Autodesk Inventor part; units mm, degrees
(part 2 of 2)
  spline S148 degree 2 poles (56.4799, 7.905) (55.3529, 7.905) (54.1022, 9.21) (54.1022, 10.347) knots 0 0 0 1 2 2 2
  spline S149 degree 2 poles (54.1022, 10.347) (54.1022, 11.4938) (55.3529, 12.7939) (56.4799, 12.7939) knots 0 0 0 1 2 2 2
  spline S150 degree 2 poles (56.4799, 12.7939) (57.607, 12.7939) (58.8527, 11.4889) (58.8527, 10.347) knots 0 0 0 1 2 2 2
  spline S151 degree 2 poles (57.3845, 10.3371) (57.3845, 10.7474) (57.2511, 11.2961) (57.1324, 11.4592) knots 0 0 0 1 2 2 2
  spline S152 degree 2 poles (57.1324, 11.4592) (57.0039, 11.6322) (56.6826, 11.7657) (56.4799, 11.7657) knots 0 0 0 1 2 2 2
  spline S153 degree 2 poles (56.4799, 11.7657) (56.2822, 11.7657) (55.9708, 11.6471) (55.8422, 11.479) knots 0 0 0 1 2 2 2
  spline S154 degree 2 poles (55.8422, 11.479) (55.7187, 11.3208) (55.5704, 10.7622) (55.5704, 10.3371) knots 0 0 0 1 2 2 2
  spline S155 degree 2 poles (55.5704, 10.3371) (55.5704, 9.9169) (55.7088, 9.3979) (55.8225, 9.2397) knots 0 0 0 1 2 2 2
  spline S156 degree 2 poles (55.8225, 9.2397) (55.9362, 9.0815) (56.2822, 8.9332) (56.4898, 8.9332) knots 0 0 0 1 2 2 2
  spline S157 degree 2 poles (56.4898, 8.9332) (56.6628, 8.9332) (57.0187, 9.0815) (57.1275, 9.2298) knots 0 0 0 1 2 2 2
  spline S158 degree 2 poles (57.1275, 9.2298) (57.2511, 9.4028) (57.3845, 9.9021) (57.3845, 10.3371) knots 0 0 0 1 2 2 2
  line L157 (63.9195, 8.0483) -> (62.4761, 8.0483)
  line L158 (62.4761, 8.0483) -> (62.4761, 10.3272)
  spline S159 degree 2 poles (62.4761, 10.3272) (62.4761, 10.609) (62.4316, 11.1626) (62.3723, 11.2911) knots 0 0 0 1 2 2 2
  spline S160 degree 2 poles (62.3723, 11.2911) (62.2982, 11.4493) (62.0213, 11.5828) (61.7841, 11.5828) knots 0 0 0 1 2 2 2
  spline S161 degree 2 poles (61.7841, 11.5828) (61.611, 11.5828) (61.2502, 11.4493) (61.0475, 11.306) knots 0 0 0 1 2 2 2
  line L159 (61.0475, 11.306) -> (61.0475, 8.0483)
  line L160 (61.0475, 8.0483) -> (59.614, 8.0483)
  line L161 (59.614, 8.0483) -> (59.614, 12.6505)
  line L162 (59.614, 12.6505) -> (61.0475, 12.6505)
  line L163 (61.0475, 12.6505) -> (61.0475, 12.1414)
  spline S162 degree 2 poles (61.0475, 12.1414) (61.3985, 12.438) (62.0658, 12.7741) (62.4712, 12.7741) knots 0 0 0 1 2 2 2
  spline S163 degree 2 poles (62.4712, 12.7741) (63.1731, 12.7741) (63.9195, 11.8843) (63.9195, 11.044) knots 0 0 0 1 2 2 2
  line L164 (63.9195, 11.044) -> (63.9195, 8.0483)
  spline S164 degree 2 poles (67.3403, 7.9248) (66.0353, 7.9248) (64.6462, 9.1705) (64.6462, 10.3223) knots 0 0 0 1 2 2 2
  spline S165 degree 2 poles (64.6462, 10.3223) (64.6462, 11.4493) (65.9413, 12.7939) (67.108, 12.7939) knots 0 0 0 1 2 2 2
  spline S166 degree 2 poles (67.108, 12.7939) (68.1609, 12.7939) (69.2286, 11.652) (69.2286, 10.5941) knots 0 0 0 1 2 2 2
  line L165 (69.2286, 10.5941) -> (69.2286, 10.0751)
  line L166 (69.2286, 10.0751) -> (66.0798, 10.0751)
  spline S167 degree 2 poles (66.0798, 10.0751) (66.0995, 9.7538) (66.3319, 9.3287) (66.5197, 9.2001) knots 0 0 0 1 2 2 2
  spline S168 degree 2 poles (66.5197, 9.2001) (66.7026, 9.0716) (67.1969, 8.9629) (67.4886, 8.9629) knots 0 0 0 1 2 2 2
  spline S169 degree 2 poles (67.4886, 8.9629) (67.7358, 8.9629) (68.2202, 9.0716) (68.4229, 9.1655) knots 0 0 0 1 2 2 2
  spline S170 degree 2 poles (68.4229, 9.1655) (68.6008, 9.2397) (68.8974, 9.4226) (68.9913, 9.4918) knots 0 0 0 1 2 2 2
  line L167 (68.9913, 9.4918) -> (69.1446, 9.4918)
  line L168 (69.1446, 9.4918) -> (69.1446, 8.3054)
  spline S171 degree 2 poles (69.1446, 8.3054) (68.9666, 8.2362) (68.6799, 8.1176) (68.4229, 8.0582) knots 0 0 0 1 2 2 2
  spline S172 degree 2 poles (68.4229, 8.0582) (68.1905, 7.994) (67.6962, 7.9248) (67.3403, 7.9248) knots 0 0 0 1 2 2 2
  spline S173 degree 2 poles (67.8148, 10.9402) (67.805, 11.3949) (67.4046, 11.8744) (66.9943, 11.8744) knots 0 0 0 1 2 2 2
  spline S174 degree 2 poles (66.9943, 11.8744) (66.5741, 11.8744) (66.0995, 11.3702) (66.0748, 10.9402) knots 0 0 0 1 2 2 2
  line L169 (66.0748, 10.9402) -> (67.8148, 10.9402)
  spline S175 degree 2 poles (71.3641, 7.9248) (70.8599, 7.9248) (69.9553, 8.1472) (69.6587, 8.2955) knots 0 0 0 1 2 2 2
  line L170 (69.6587, 8.2955) -> (69.6587, 9.5066)
  line L171 (69.6587, 9.5066) -> (69.7773, 9.5066)
  spline S176 degree 2 poles (69.7773, 9.5066) (69.8811, 9.4275) (70.1431, 9.2397) (70.3755, 9.1359) knots 0 0 0 1 2 2 2
  spline S177 degree 2 poles (70.3755, 9.1359) (70.5781, 9.0419) (71.0774, 8.9085) (71.374, 8.9085) knots 0 0 0 1 2 2 2
  spline S178 degree 2 poles (71.374, 8.9085) (71.6755, 8.9085) (72.1402, 9.0963) (72.1402, 9.299) knots 0 0 0 1 2 2 2
  spline S179 degree 2 poles (72.1402, 9.299) (72.1402, 9.4572) (71.9277, 9.6253) (71.6212, 9.6945) knots 0 0 0 1 2 2 2
  spline S180 degree 2 poles (71.6212, 9.6945) (71.458, 9.7389) (70.9588, 9.8329) (70.766, 9.8922) knots 0 0 0 1 2 2 2
  spline S181 degree 2 poles (70.766, 9.8922) (70.2222, 10.0603) (69.6785, 10.7177) (69.6785, 11.2565) knots 0 0 0 1 2 2 2
  spline S182 degree 2 poles (69.6785, 11.2565) (69.6785, 11.563) (69.9602, 12.1068) (70.2371, 12.3193) knots 0 0 0 1 2 2 2
  spline S183 degree 2 poles (70.2371, 12.3193) (70.5089, 12.527) (71.3147, 12.7741) (71.8238, 12.7741) knots 0 0 0 1 2 2 2
  spline S184 degree 2 poles (71.8238, 12.7741) (72.3083, 12.7741) (73.119, 12.5813) (73.3958, 12.4479) knots 0 0 0 1 2 2 2
  line L172 (73.3958, 12.4479) -> (73.3958, 11.2812)
  line L173 (73.3958, 11.2812) -> (73.2821, 11.2812)
  spline S185 degree 2 poles (73.2821, 11.2812) (73.208, 11.3406) (72.8866, 11.5334) (72.7384, 11.6026) knots 0 0 0 1 2 2 2
  spline S186 degree 2 poles (72.7384, 11.6026) (72.5554, 11.6817) (72.1106, 11.7904) (71.8782, 11.7904) knots 0 0 0 1 2 2 2
  spline S187 degree 2 poles (71.8782, 11.7904) (71.5668, 11.7904) (71.1367, 11.5778) (71.1367, 11.4048) knots 0 0 0 1 2 2 2
  spline S188 degree 2 poles (71.1367, 11.4048) (71.1367, 11.2466) (71.3493, 11.0687) (71.7052, 10.9797) knots 0 0 0 1 2 2 2
  spline S189 degree 2 poles (71.7052, 10.9797) (71.8881, 10.9352) (72.3676, 10.8512) (72.5901, 10.777) knots 0 0 0 1 2 2 2
  spline S190 degree 2 poles (72.5901, 10.777) (73.0844, 10.6189) (73.5985, 10.0009) (73.5985, 9.4868) knots 0 0 0 1 2 2 2
  spline S191 degree 2 poles (73.5985, 9.4868) (73.5985, 9.1655) (73.2969, 8.5773) (73.0152, 8.3795) knots 0 0 0 1 2 2 2
  spline S192 degree 2 poles (73.0152, 8.3795) (72.7235, 8.162) (71.9227, 7.9248) (71.3641, 7.9248) knots 0 0 0 1 2 2 2
  line L174 (75.7142, 8.0483) -> (74.2807, 8.0483)
  line L175 (74.2807, 8.0483) -> (74.2807, 12.6505)
  line L176 (74.2807, 12.6505) -> (75.7142, 12.6505)
  line L177 (75.7142, 12.6505) -> (75.7142, 8.0483)
  line L178 (75.7587, 13.308) -> (74.2411, 13.308)
  line L179 (74.2411, 13.308) -> (74.2411, 14.4252)
  line L180 (74.2411, 14.4252) -> (75.7587, 14.4252)
  line L181 (75.7587, 14.4252) -> (75.7587, 13.308)
  spline S193 degree 2 poles (79.3475, 8.5377) (79.1992, 8.4142) (78.9669, 8.2164) (78.7691, 8.1176) knots 0 0 0 1 2 2 2
  spline S194 degree 2 poles (78.7691, 8.1176) (78.5764, 8.0236) (78.2106, 7.9248) (77.8843, 7.9248) knots 0 0 0 1 2 2 2
  spline S195 degree 2 poles (77.8843, 7.9248) (77.2713, 7.9248) (76.4656, 8.7453) (76.4656, 9.3682) knots 0 0 0 1 2 2 2
  spline S196 degree 2 poles (76.4656, 9.3682) (76.4656, 9.8774) (76.8759, 10.5101) (77.2614, 10.693) knots 0 0 0 1 2 2 2
  spline S197 degree 2 poles (77.2614, 10.693) (77.652, 10.8808) (78.7345, 11.0291) (79.3574, 11.0687) knots 0 0 0 1 2 2 2
  line L182 (79.3574, 11.0687) -> (79.3574, 11.0934)
  spline S198 degree 2 poles (79.3574, 11.0934) (79.3574, 11.474) (78.7939, 11.7657) (78.2303, 11.7657) knots 0 0 0 1 2 2 2
  spline S199 degree 2 poles (78.2303, 11.7657) (77.9782, 11.7657) (77.296, 11.5828) (76.9747, 11.4394) knots 0 0 0 1 2 2 2
  line L183 (76.9747, 11.4394) -> (76.8512, 11.4394)
  line L184 (76.8512, 11.4394) -> (76.8512, 12.5517)
  spline S200 degree 2 poles (76.8512, 12.5517) (77.0637, 12.611) (78.0128, 12.7791) (78.4973, 12.7791) knots 0 0 0 1 2 2 2
  spline S201 degree 2 poles (78.4973, 12.7791) (79.6837, 12.7791) (80.7712, 11.9881) (80.7712, 11.1774) knots 0 0 0 1 2 2 2
  line L185 (80.7712, 11.1774) -> (80.7712, 8.0483)
  line L186 (80.7712, 8.0483) -> (79.3475, 8.0483)
  line L187 (79.3475, 8.0483) -> (79.3475, 8.5377)
  line L188 (79.3475, 9.2496) -> (79.3475, 10.2036)
  spline S202 degree 2 poles (79.3475, 10.2036) (78.9817, 10.169) (78.5319, 10.1146) (78.3144, 10.0355) knots 0 0 0 1 2 2 2
  spline S203 degree 2 poles (78.3144, 10.0355) (78.1216, 9.9713) (77.914, 9.7043) (77.914, 9.4868) knots 0 0 0 1 2 2 2
  spline S204 degree 2 poles (77.914, 9.4868) (77.914, 9.1655) (78.2649, 8.9233) (78.606, 8.9233) knots 0 0 0 1 2 2 2
  spline S205 degree 2 poles (78.606, 8.9233) (78.7939, 8.9233) (79.1893, 9.0963) (79.3475, 9.2496) knots 0 0 0 1 2 2 2
  point P0 (60.406, 3)
  constraints: 2 other
extrude "Extrusion36" cut sketch "Sketch38" against normal blind 2
sketch "Sketch39" plane through (-60.406, -3, -27.1071) normal (-1, 0, 0) x (0, 0, 1)
  circle A0 centre (3, 31.508) radius 1
  circle A1 centre (3, 20.723) radius 1
  line L0 (0, 63) -> (0, 17.2226) projected
  line L1 (54.2141, 0) -> (0, 0) projected
  point P0 (27.1071, 3)
  dimension "d265" = 2
  dimension "d266" = 2
  dimension "d267" = 3
  dimension "d268" = 3
  dimension "d269" = 10.785
  dimension "d270" = 20.723
  constraints: 2 centre point
  measures "d265" diameter of A0
  measures "d266" diameter of A1
  measures "d267" distance from line of A0.centre L0
  measures "d268" distance from line of L0 A1.centre
  measures "d269" distance of A1.centre A0.centre
  measures "d270" distance from line of A1.centre L1
extrude "Extrusion37" cut sketch "Sketch39" against normal through all
sketch "Sketch40" plane through (0, 0, 0) normal (0, 1, 0) x (1, 0, 0)
  circle A0 centre (37.593, -4.5441) radius 1.75 projected
  circle A1 centre (32.8575, -4.3056) radius 1.75 projected
  circle A2 centre (-32.8575, -4.3056) radius 1.75 projected
  circle A3 centre (-37.593, -4.5441) radius 1.75 projected
  circle A4 centre (37.593, 0.2259) radius 1.75
  circle A5 centre (32.8575, 0.4644) radius 1.75
  circle A6 centre (37.593, 4.9959) radius 1.75
  circle A7 centre (32.8575, 5.2344) radius 1.75
  circle A8 centre (-37.593, 0.2259) radius 1.75
  circle A9 centre (-32.8575, 0.4644) radius 1.75
  circle A10 centre (-37.593, 4.9959) radius 1.75
  circle A11 centre (-32.8575, 5.2344) radius 1.75
  line L0 (29.3575, -7.2941) -> (-29.3575, -7.2941) projected
  line L1 (29.3575, 12.7544) -> (-29.3575, 12.7544)
  line L2 (-29.3575, 4.6829) -> (29.3575, 4.6829) projected
  line L3 (29.3575, 12.7544) -> (29.3575, 4.6829)
  line L4 (-29.3575, 12.7544) -> (-29.3575, 4.6829)
  circle A12 centre (37.593, 9.7659) radius 1.75
  circle A13 centre (32.8575, 10.0044) radius 1.75
  circle A14 centre (-37.593, 9.7659) radius 1.75
  circle A15 centre (-32.8575, 10.0044) radius 1.75
  point P0 (0, 0)
  dimension "d273" = 3.5
  dimension "d274" = 3.5
  dimension "d275" = 4.7355
  dimension "d276" = 0.2385
  dimension "d277" = 0.2385
  dimension "d278" = 4.77
  dimension "d279" = 3.5
  dimension "d280" = 3.5
  dimension "d281" = 0.2385
  dimension "d283" = 4.77
  dimension "d284" = 2.9885
  dimension "d298" = 4.77
  dimension "d301" = 2.9885
  constraints: 12 centre point, 6 end point, 6 vertical alignment, 1 horizontal, 1 parallel, 1 vertical
  measures "d273" diameter of A4
  measures "d274" diameter of A5
  measures "d275" horizontal distance of A1.centre A0.centre
  measures "d276" vertical distance of A1.centre A0.centre
  measures "d277" vertical distance of A5.centre A4.centre
  measures "d278" distance of A5.centre A1.centre
  measures "d279" diameter of A6
  measures "d280" diameter of A7
  measures "d281" vertical distance of A7.centre A6.centre
  measures "d283" distance of A7.centre A5.centre
  measures "d284" distance from line of A1.centre L0
  measures "d298" distance of A12.centre A6.centre
  measures "d301" distance from line of A12.centre L1
extrude "Extrusion38" cut sketch "Sketch40" against normal through all contours A4 | A5 | A6 | A7 | A8 | A9 | A10 | A11 | L3 L2 L4 L1
extrude "Extrusion39" cut sketch "Sketch40" against normal through all contours A12 | A13 | A14 | A15
sketch "Sketch41" plane through (28.495, 37.5, 27.1071) normal (0, 1, 0) x (1, 0, 0)
  line L0 (17.2371, -0.591) -> (19.0325, -0.591) construction
  line L1 (19.0325, -0.591) -> (19.0325, -4.091) construction
  line L2 (19.0325, -4.091) -> (17.2371, -4.091) construction
  line L3 (17.2371, -4.091) -> (17.2371, -0.591) construction
  line L4 (0.3973, -0.7222) -> (2.8059, -0.7222) construction
  line L5 (2.8059, -0.7222) -> (2.8059, -4.3665) construction
  line L6 (2.8059, -4.3665) -> (0.3973, -4.3665) construction
  line L7 (0.3973, -4.3665) -> (0.3973, -0.7222) construction
  line L8 (-28.495, 27.1071) -> (-28.495, -17)
  spline S0 degree 2 poles (2.6904, -2.8343) (2.6904, -3.3486) (2.6406, -3.7946) (2.3704, -4.1671) (1.9191, -4.3665) (1.62, -4.3665) knots 0 0 0 1 2 3 4 4 4
  spline S1 degree 2 poles (1.62, -4.3665) (1.3366, -4.3665) (0.8801, -4.1803) (0.602, -3.8024) (0.5495, -3.3669) (0.5495, -2.8343) knots 0 0 0 1 2 3 4 4 4
  line L9 (0.5495, -2.8343) -> (0.5495, -2.2518)
  spline S2 degree 2 poles (0.5495, -2.2518) (0.5495, -1.7324) (0.5994, -1.2942) (0.867, -0.9216) (1.3235, -0.7222) (1.62, -0.7222) knots 0 0 0 1 2 3 4 4 4
  spline S3 degree 2 poles (1.62, -0.7222) (1.9033, -0.7222) (2.3599, -0.9111) (2.638, -1.2863) (2.6904, -1.7245) (2.6904, -2.2518) knots 0 0 0 1 2 3 4 4 4
  line L10 (2.6904, -2.2518) -> (2.6904, -2.8343)
  spline S4 degree 2 poles (1.7144, -1.714) (1.7144, -1.4831) (1.6751, -1.386) (1.6252, -1.386) knots 0 0 0 1 2 2 2
  spline S5 degree 2 poles (1.6252, -1.386) (1.578, -1.386) (1.5255, -1.4621) (1.5255, -1.714) knots 0 0 0 1 2 2 2
  line L11 (1.5255, -1.714) -> (1.5255, -3.3092)
  spline S6 degree 2 poles (1.5255, -3.3092) (1.5255, -3.6004) (1.5623, -3.7027) (1.6174, -3.7027) knots 0 0 0 1 2 2 2
  spline S7 degree 2 poles (1.6174, -3.7027) (1.6751, -3.7027) (1.7144, -3.5768) (1.7144, -3.283) knots 0 0 0 1 2 2 2
  line L12 (1.7144, -3.283) -> (1.7144, -1.714)
  line L13 (2.9843, -0.7957) -> (4.5769, -0.7957)
  line L14 (4.5769, -0.7957) -> (4.5769, -1.5644)
  line L15 (4.5769, -1.5644) -> (3.9603, -1.5644)
  line L16 (3.9603, -1.5644) -> (3.9603, -2.1233)
  line L17 (3.9603, -2.1233) -> (4.5087, -2.1233)
  line L18 (4.5087, -2.1233) -> (4.5087, -2.8605)
  line L19 (4.5087, -2.8605) -> (3.9603, -2.8605)
  line L20 (3.9603, -2.8605) -> (3.9603, -4.2957)
  line L21 (3.9603, -4.2957) -> (2.9843, -4.2957)
  line L22 (2.9843, -4.2957) -> (2.9843, -0.7957)
  line L23 (4.7395, -0.7957) -> (6.3321, -0.7957)
  line L24 (6.3321, -0.7957) -> (6.3321, -1.5644)
  line L25 (6.3321, -1.5644) -> (5.7156, -1.5644)
  line L26 (5.7156, -1.5644) -> (5.7156, -2.1233)
  line L27 (5.7156, -2.1233) -> (6.2639, -2.1233)
  line L28 (6.2639, -2.1233) -> (6.2639, -2.8605)
  line L29 (6.2639, -2.8605) -> (5.7156, -2.8605)
  line L30 (5.7156, -2.8605) -> (5.7156, -4.2957)
  line L31 (5.7156, -4.2957) -> (4.7395, -4.2957)
  line L32 (4.7395, -4.2957) -> (4.7395, -0.7957)
  spline S8 degree 2 poles (19.5302, -2.7031) (19.5302, -3.2173) (19.4804, -3.6633) (19.2101, -4.0359) (18.7588, -4.2353) (18.4597, -4.2353) knots 0 0 0 1 2 3 4 4 4
  spline S9 degree 2 poles (18.4597, -4.2353) (18.1764, -4.2353) (17.7199, -4.049) (17.4418, -3.6712) (17.3893, -3.2357) (17.3893, -2.7031) knots 0 0 0 1 2 3 4 4 4
  line L33 (17.3893, -2.7031) -> (17.3893, -2.1206)
  spline S10 degree 2 poles (17.3893, -2.1206) (17.3893, -1.6011) (17.4391, -1.163) (17.7067, -0.7904) (18.1633, -0.591) (18.4597, -0.591) knots 0 0 0 1 2 3 4 4 4
  spline S11 degree 2 poles (18.4597, -0.591) (18.7431, -0.591) (19.1996, -0.7799) (19.4777, -1.1551) (19.5302, -1.5932) (19.5302, -2.1206) knots 0 0 0 1 2 3 4 4 4
  line L34 (19.5302, -2.1206) -> (19.5302, -2.7031)
  spline S12 degree 2 poles (18.5542, -1.5827) (18.5542, -1.3519) (18.5148, -1.2548) (18.465, -1.2548) knots 0 0 0 1 2 2 2
  spline S13 degree 2 poles (18.465, -1.2548) (18.4178, -1.2548) (18.3653, -1.3309) (18.3653, -1.5827) knots 0 0 0 1 2 2 2
  line L35 (18.3653, -1.5827) -> (18.3653, -3.1779)
  spline S14 degree 2 poles (18.3653, -3.1779) (18.3653, -3.4692) (18.402, -3.5715) (18.4571, -3.5715) knots 0 0 0 1 2 2 2
  spline S15 degree 2 poles (18.4571, -3.5715) (18.5148, -3.5715) (18.5542, -3.4456) (18.5542, -3.1517) knots 0 0 0 1 2 2 2
  line L36 (18.5542, -3.1517) -> (18.5542, -1.5827)
  line L37 (21.8942, -0.6645) -> (21.8942, -4.1645)
  line L38 (21.8942, -4.1645) -> (21.0388, -4.1645)
  line L39 (21.0388, -4.1645) -> (20.6558, -2.6139)
  line L40 (20.6558, -2.6139) -> (20.6558, -4.1645)
  line L41 (20.6558, -4.1645) -> (19.8241, -4.1645)
  line L42 (19.8241, -4.1645) -> (19.8241, -0.6645)
  line L43 (19.8241, -0.6645) -> (20.64, -0.6645)
  line L44 (20.64, -0.6645) -> (21.0624, -2.1993)
  line L45 (21.0624, -2.1993) -> (21.0624, -0.6645)
  line L46 (21.0624, -0.6645) -> (21.8942, -0.6645)
  constraints: 2 end point, 2 horizontal, 1 vertical, 4 other
extrude "Extrusion40" cut sketch "Sketch41" against normal through all
sketch "Sketch42" plane through (30.0205, 37.5, 30.4163) normal (0, 1, 0) x (1, 0, 0)
  spline S0 degree 2 poles (0.0997, 1.9232) (0.0525, 1.9232) (0, 1.8471) (0, 1.5952) knots 0 0 0 0.5 1 1 1 projected
  line L0 (0, 1.5952) -> (0, 0) projected
  spline S1 degree 2 poles (0, 0) (0, -0.2912) (0.0367, -0.3936) (0.0918, -0.3936) knots 0 0 0 0.5 1 1 1 projected
  spline S2 degree 2 poles (0.0918, -0.3936) (0.1496, -0.3936) (0.1889, -0.2676) (0.1889, 0.0262) knots 0 0 0 0.5 1 1 1 projected
  line L1 (0.1889, 0.0262) -> (0.1889, 1.5952) projected
  spline S3 degree 2 poles (0.1889, 1.5952) (0.1889, 1.8261) (0.1496, 1.9232) (0.0997, 1.9232) knots 0 0 0 0.5 1 1 1 projected
  point P0 (-30.0205, 30.4163)
  constraints: 4 other
extrude "Extrusion41" cut sketch "Sketch42" against normal through all
sketch "Sketch43" plane through (28.495, 37.5, 27.1071) normal (0, 1, 0) x (1, 0, 0)
  spline S0 degree 2 poles (18.465, -1.2548) (18.4178, -1.2548) (18.3653, -1.3309) (18.3653, -1.5827) knots 0 0 0 0.5 1 1 1 projected
  line L0 (18.3653, -1.5827) -> (18.3653, -3.1779) projected
  spline S1 degree 2 poles (18.3653, -3.1779) (18.3653, -3.4692) (18.402, -3.5715) (18.4571, -3.5715) knots 0 0 0 0.5 1 1 1 projected
  spline S2 degree 2 poles (18.4571, -3.5715) (18.5148, -3.5715) (18.5542, -3.4456) (18.5542, -3.1517) knots 0 0 0 0.5 1 1 1 projected
  line L1 (18.5542, -3.1517) -> (18.5542, -1.5827) projected
  spline S3 degree 2 poles (18.5542, -1.5827) (18.5542, -1.3519) (18.5148, -1.2548) (18.465, -1.2548) knots 0 0 0 0.5 1 1 1 projected
  point P0 (-28.495, 27.1071)
  constraints: 4 other
extrude "Extrusion42" cut sketch "Sketch43" against normal through all
sketch "Sketch44" plane through (-50.995, 37.5, 27.1071) normal (0, 1, 0) x (1, 0, 0)
  line L0 (15.9264, -0.607) -> (21.8454, -0.607) construction
  line L1 (21.8454, -0.607) -> (21.8454, -4.2513) construction
  line L2 (21.8454, -4.2513) -> (15.9264, -4.2513) construction
  line L3 (15.9264, -4.2513) -> (15.9264, -0.607) construction
  line L4 (0.8421, -0.8846) -> (5.6382, -0.8846) construction
  line L5 (5.6382, -0.8846) -> (5.6382, -4.5289) construction
  line L6 (5.6382, -4.5289) -> (0.8421, -4.5289) construction
  line L7 (0.8421, -4.5289) -> (0.8421, -0.8846) construction
  spline S0 degree 2 poles (3.1352, -2.9967) (3.1352, -3.5109) (3.0854, -3.957) (2.8152, -4.3295) (2.3639, -4.5289) (2.0648, -4.5289) knots 0 0 0 1 2 3 4 4 4
  spline S1 degree 2 poles (2.0648, -4.5289) (1.7814, -4.5289) (1.3249, -4.3426) (1.0468, -3.9648) (0.9943, -3.5293) (0.9943, -2.9967) knots 0 0 0 1 2 3 4 4 4
  line L8 (0.9943, -2.9967) -> (0.9943, -2.4142)
  spline S2 degree 2 poles (0.9943, -2.4142) (0.9943, -1.8947) (1.0442, -1.4566) (1.3118, -1.084) (1.7683, -0.8846) (2.0648, -0.8846) knots 0 0 0 1 2 3 4 4 4
  spline S3 degree 2 poles (2.0648, -0.8846) (2.3481, -0.8846) (2.8047, -1.0735) (3.0828, -1.4487) (3.1352, -1.8869) (3.1352, -2.4142) knots 0 0 0 1 2 3 4 4 4
  line L9 (3.1352, -2.4142) -> (3.1352, -2.9967)
  spline S4 degree 2 poles (2.1592, -1.8764) (2.1592, -1.6455) (2.1199, -1.5484) (2.07, -1.5484) knots 0 0 0 1 2 2 2
  spline S5 degree 2 poles (2.07, -1.5484) (2.0228, -1.5484) (1.9703, -1.6245) (1.9703, -1.8764) knots 0 0 0 1 2 2 2
  line L10 (1.9703, -1.8764) -> (1.9703, -3.4716)
  spline S6 degree 2 poles (1.9703, -3.4716) (1.9703, -3.7628) (2.0071, -3.8651) (2.0622, -3.8651) knots 0 0 0 1 2 2 2
  spline S7 degree 2 poles (2.0622, -3.8651) (2.1199, -3.8651) (2.1592, -3.7392) (2.1592, -3.4453) knots 0 0 0 1 2 2 2
  line L11 (2.1592, -3.4453) -> (2.1592, -1.8764)
  line L12 (5.4992, -0.9581) -> (5.4992, -4.4581)
  line L13 (5.4992, -4.4581) -> (4.6439, -4.4581)
  line L14 (4.6439, -4.4581) -> (4.2608, -2.9075)
  line L15 (4.2608, -2.9075) -> (4.2608, -4.4581)
  line L16 (4.2608, -4.4581) -> (3.4291, -4.4581)
  line L17 (3.4291, -4.4581) -> (3.4291, -0.9581)
  line L18 (3.4291, -0.9581) -> (4.2451, -0.9581)
  line L19 (4.2451, -0.9581) -> (4.6675, -2.4929)
  line L20 (4.6675, -2.4929) -> (4.6675, -0.9581)
  line L21 (4.6675, -0.9581) -> (5.4992, -0.9581)
  spline S8 degree 2 poles (18.2195, -2.7191) (18.2195, -3.2333) (18.1696, -3.6793) (17.8994, -4.0519) (17.4481, -4.2513) (17.149, -4.2513) knots 0 0 0 1 2 3 4 4 4
  spline S9 degree 2 poles (17.149, -4.2513) (16.8657, -4.2513) (16.4091, -4.065) (16.131, -3.6872) (16.0786, -3.2517) (16.0786, -2.7191) knots 0 0 0 1 2 3 4 4 4
  line L22 (16.0786, -2.7191) -> (16.0786, -2.1366)
  spline S10 degree 2 poles (16.0786, -2.1366) (16.0786, -1.6171) (16.1284, -1.179) (16.396, -0.8064) (16.8525, -0.607) (17.149, -0.607) knots 0 0 0 1 2 3 4 4 4
  spline S11 degree 2 poles (17.149, -0.607) (17.4324, -0.607) (17.8889, -0.7959) (18.167, -1.1711) (18.2195, -1.6092) (18.2195, -2.1366) knots 0 0 0 1 2 3 4 4 4
  line L23 (18.2195, -2.1366) -> (18.2195, -2.7191)
  spline S12 degree 2 poles (17.2435, -1.5987) (17.2435, -1.3679) (17.2041, -1.2708) (17.1543, -1.2708) knots 0 0 0 1 2 2 2
  spline S13 degree 2 poles (17.1543, -1.2708) (17.107, -1.2708) (17.0546, -1.3469) (17.0546, -1.5987) knots 0 0 0 1 2 2 2
  line L24 (17.0546, -1.5987) -> (17.0546, -3.1939)
  spline S14 degree 2 poles (17.0546, -3.1939) (17.0546, -3.4852) (17.0913, -3.5875) (17.1464, -3.5875) knots 0 0 0 1 2 2 2
  spline S15 degree 2 poles (17.1464, -3.5875) (17.2041, -3.5875) (17.2435, -3.4616) (17.2435, -3.1677) knots 0 0 0 1 2 2 2
  line L25 (17.2435, -3.1677) -> (17.2435, -1.5987)
  line L26 (18.5133, -0.6805) -> (20.1059, -0.6805)
  line L27 (20.1059, -0.6805) -> (20.1059, -1.4492)
  line L28 (20.1059, -1.4492) -> (19.4893, -1.4492)
  line L29 (19.4893, -1.4492) -> (19.4893, -2.008)
  line L30 (19.4893, -2.008) -> (20.0377, -2.008)
  line L31 (20.0377, -2.008) -> (20.0377, -2.7453)
  line L32 (20.0377, -2.7453) -> (19.4893, -2.7453)
  line L33 (19.4893, -2.7453) -> (19.4893, -4.1805)
  line L34 (19.4893, -4.1805) -> (18.5133, -4.1805)
  line L35 (18.5133, -4.1805) -> (18.5133, -0.6805)
  line L36 (20.2686, -0.6805) -> (21.8612, -0.6805)
  line L37 (21.8612, -0.6805) -> (21.8612, -1.4492)
  line L38 (21.8612, -1.4492) -> (21.2446, -1.4492)
  line L39 (21.2446, -1.4492) -> (21.2446, -2.008)
  line L40 (21.2446, -2.008) -> (21.7929, -2.008)
  line L41 (21.7929, -2.008) -> (21.7929, -2.7453)
  line L42 (21.7929, -2.7453) -> (21.2446, -2.7453)
  line L43 (21.2446, -2.7453) -> (21.2446, -4.1805)
  line L44 (21.2446, -4.1805) -> (20.2686, -4.1805)
  line L45 (20.2686, -4.1805) -> (20.2686, -0.6805)
  point P0 (50.995, 27.1071)
  constraints: 4 other
extrude "Extrusion43" cut sketch "Sketch44" against normal through all
sketch "Sketch45" plane through (-50.995, 37.5, 27.1071) normal (0, 1, 0) x (1, 0, 0)
  spline S0 degree 2 poles (2.07, -1.5484) (2.0228, -1.5484) (1.9703, -1.6245) (1.9703, -1.8764) knots 0 0 0 0.5 1 1 1 projected
  line L0 (1.9703, -1.8764) -> (1.9703, -3.4716) projected
  spline S1 degree 2 poles (1.9703, -3.4716) (1.9703, -3.7628) (2.0071, -3.8651) (2.0622, -3.8651) knots 0 0 0 0.5 1 1 1 projected
  spline S2 degree 2 poles (2.0622, -3.8651) (2.1199, -3.8651) (2.1592, -3.7392) (2.1592, -3.4453) knots 0 0 0 0.5 1 1 1 projected
  line L1 (2.1592, -3.4453) -> (2.1592, -1.8764) projected
  spline S3 degree 2 poles (2.1592, -1.8764) (2.1592, -1.6455) (2.1199, -1.5484) (2.07, -1.5484) knots 0 0 0 0.5 1 1 1 projected
  spline S4 degree 2 poles (17.1543, -1.2708) (17.107, -1.2708) (17.0546, -1.3469) (17.0546, -1.5987) knots 0 0 0 0.5 1 1 1 projected
  line L2 (17.0546, -1.5987) -> (17.0546, -3.1939) projected
  spline S5 degree 2 poles (17.0546, -3.1939) (17.0546, -3.4852) (17.0913, -3.5875) (17.1464, -3.5875) knots 0 0 0 0.5 1 1 1 projected
  spline S6 degree 2 poles (17.1464, -3.5875) (17.2041, -3.5875) (17.2435, -3.4616) (17.2435, -3.1677) knots 0 0 0 0.5 1 1 1 projected
  line L3 (17.2435, -3.1677) -> (17.2435, -1.5987) projected
  spline S7 degree 2 poles (17.2435, -1.5987) (17.2435, -1.3679) (17.2041, -1.2708) (17.1543, -1.2708) knots 0 0 0 0.5 1 1 1 projected
  point P0 (50.995, 27.1071)
  constraints: 8 other
extrude "Extrusion44" cut sketch "Sketch45" against normal through all
equation "\"d249\" = 0.5 * d248"
equation "\"d243\" = 0.5 * d242"
equation "\"d255\" = d254"
body "Solid2"
